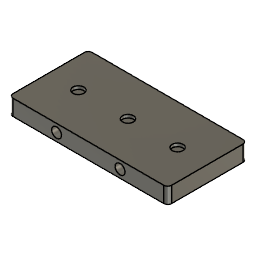
Base (Autodesk Fusion 360 design; units mm, degrees)
part number: 2026-03-04-09-38-15-257
Autodesk Fusion 360 part; units mm, degrees
sketch "Sketch1" plane through (0, 0, 0) normal (0, 0, 1) x (1, 0, 0)
  line L0 (50.8, -25.4) -> (-50.8, -25.4)
  line L1 (-50.8, -25.4) -> (-50.8, 25.4)
  line L2 (-50.8, 25.4) -> (50.8, 25.4)
  line L3 (50.8, 25.4) -> (50.8, -25.4)
  line L4 (50.8, -25.4) -> (-50.8, 25.4) construction
  line L5 (-50.8, -25.4) -> (50.8, 25.4) construction
  dimension "d2" = 101.6
  dimension "d8" = 50.8
  constraint horizontal L0
  constraint perpendicular L0 L1
  constraint parallel L0 L2
  constraint parallel L1 L3
  constraint coincident L4 origin
  constraint coincident L5 origin
  measures "d2" distance of L1 L3
  measures "d8" distance of L0 L2
extrude "Extrude1" add sketch "Sketch1" against normal blind 10.16
sketch "Sketch2" plane through (0, 0, 0) normal (0, 0, 1) x (-1, 0, 0)
  line L0 (-50.8, -25.4) -> (50.8, -25.4)
  line L1 (50.8, -25.4) -> (50.8, 25.4)
  line L2 (50.8, 25.4) -> (-50.8, 25.4)
  line L3 (-50.8, 25.4) -> (-50.8, -25.4)
  circle A0 centre (31.75, 0) radius 3.5
  circle A1 centre (0, 0) radius 3.5
  circle A2 centre (-31.75, 0) radius 3.5
  line L4 (12.7, -25.4) -> (12.7, 25.4) construction
  dimension "d11" = 7
  dimension "d12" = 19.05
  dimension "d13" = 7
  dimension "d14" = 50.8
  dimension "d15" = 7
  dimension "d16" = 19.05
  dimension "d17" = 25.4
  dimension "d18" = 25.4
  dimension "d19" = 25.4
  dimension "d22" = 38.1
  constraint coincident L0 L4.start
  constraint coincident L2 L4.end
  constraint perpendicular L2 L4
  measures "d11" diameter of A0
  measures "d12" distance of L1 A0.centre
  measures "d13" diameter of A1
  measures "d14" distance of L3 A1.centre
  measures "d15" diameter of A2
  measures "d16" distance of L3 A2.centre
  measures "d17" distance of L2 A0.centre
  measures "d18" distance of L2 A1.centre
  measures "d19" distance of L2 A2.centre
  measures "d22" distance of L1 L4
extrude "Extrude2" cut sketch "Sketch2" against normal blind 2 contours A0 | A1 | A2
sketch "Sketch3" plane through (0, -25.4, 0) normal (0, -1, 0) x (1, 0, 0)
  line L0 (50.8, 0) -> (-50.8, 0)
  line L1 (-50.8, 0) -> (-50.8, -10.16)
  line L2 (-50.8, -10.16) -> (50.8, -10.16)
  line L3 (50.8, -10.16) -> (50.8, 0)
  circle A0 centre (-20.32, -5.08) radius 3.175
  circle A1 centre (20.32, -5.08) radius 3.175
  dimension "d23" = 30.48
  dimension "d24" = 30.48
  dimension "d25" = 6.35
  dimension "d26" = 6.35
  dimension "d27" = 5.08
  dimension "d28" = 5.08
  measures "d23" distance of L1 A0.centre
  measures "d24" distance of L3 A1.centre
  measures "d25" diameter of A0
  measures "d26" diameter of A1
  measures "d27" distance of L0 A0.centre
  measures "d28" distance of L0 A1.centre
extrude "Extrude3" cut sketch "Sketch3" against normal through all contours A0 | A1
fillet "Fillet1" radius 2.54 4 edges at (-50.8, -25.4, -5.08) (-50.8, 25.4, -5.08) (50.8, -25.4, -5.08) (50.8, 25.4, -5.08)
